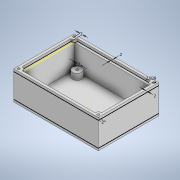
# Autodesk Inventor part: Enclosure
Saved by Autodesk Inventor 2020.2 (Build 242310000, 310)
## iProperties
Created: 2020-09-23
Part Number: Enclosure
Material: Generic
Document SubType Name: Modeling
Designer: johnf
Density: 1 g/cm^3
Appearance: Default
Author: johnf
Autodesk Inventor part; units mm, degrees
ref_plane "YZ Plane" through (0, 0, 0) normal (1, 0, 0) x (0, 1, 0)
ref_plane "XZ Plane" through (0, 0, 0) normal (0, 1, 0) x (-1, 0, 0)
ref_plane "XY Plane" through (0, 0, 0) normal (0, 0, 1) x (1, 0, 0)
sketch "Sketch1" plane through (0, 0, 0) normal (0, 1, 0) x (-1, 0, 0)
  line L0 (25, 17.5) -> (-25, 17.5) construction
  line L1 (-25, 17.5) -> (-25, -17.5) construction
  line L2 (-25, -17.5) -> (25, -17.5) construction
  line L3 (25, -17.5) -> (25, 17.5) construction
  line L4 (25, -17.5) -> (-25, 17.5) construction
  circle A0 centre (25, 17.5) radius 1
  circle A1 centre (25, -17.5) radius 1
  circle A2 centre (-25, 17.5) radius 1
  circle A3 centre (-25, -17.5) radius 1
  circle A4 centre (25, 17.5) radius 3.75
  circle A5 centre (25, -17.5) radius 3.75
  circle A6 centre (-25, -17.5) radius 3.75
  circle A7 centre (-25, 17.5) radius 3.75
  point P0 (0, 0)
  point P1 (0, 0)
  dimension "d0" = 35
  dimension "d1" = 50
  dimension "d2" = 2
  dimension "d3" = 7.5
  constraints: 10 end point, 9 coincident, 8 centre point, 6 equal radius, 2 parallel, 1 horizontal, 1 midpoint, 1 perpendicular
  measures "d0" distance of L2.end L0.start
  measures "d1" distance of L1.end L2.end
  measures "d2" diameter of A0
  measures "d3" diameter of A4
extrude "Extrusion1" add sketch "Sketch1" along normal blind 5
sketch "Sketch2" plane through (0, 0, 0) normal (0, 1, 0) x (-1, 0, 0)
  line L0 (35, -25) -> (-35, -25)
  line L1 (-35, -25) -> (-35, 25)
  line L2 (-35, 25) -> (35, 25)
  line L3 (35, 25) -> (35, -25)
  line L4 (35, 25) -> (-35, -25) construction
  line L5 (30, -22.5) -> (-30, -22.5) construction
  line L6 (-30, -22.5) -> (-30, 22.5) construction
  line L7 (-30, 22.5) -> (30, 22.5) construction
  line L8 (30, 22.5) -> (30, -22.5) construction
  line L9 (-25, -17.5) -> (25, -17.5) construction
  line L10 (25, -17.5) -> (25, 17.5) construction
  line L11 (25, 17.5) -> (-25, 17.5) construction
  line L12 (-25, 17.5) -> (-25, -17.5) construction
  line L13 (30, -22.5) -> (-30, 22.5) construction
  line L14 (-31, -21) -> (31, -21)
  line L15 (31, -21) -> (31, 21)
  line L16 (31, 21) -> (-31, 21)
  line L17 (-31, 21) -> (-31, -21)
  point P0 (0, 0)
  point P1 (0, 0)
  dimension "d6" = 70
  dimension "d7" = 60
  dimension "d8" = 45
  dimension "d9" = 5
  dimension "d10" = 50
  dimension "d11" = 4
  constraints: 36 end point, 8 parallel, 4 perpendicular, 2 horizontal, 2 midpoint, 1 coincident, 6 other
  measures "d6" distance of L0.start L0.end
  measures "d7" distance of L5.start L5.end
  measures "d8" distance of L7.end L5.start
  measures "d9" distance between parallel lines of L5 L9
  measures "d10" distance of L2.end L0.start
  measures "d11" distance between parallel lines of L3 L15
extrude "Extrusion2" add sketch "Sketch2" against normal blind 2 contours L0 L1 L2 L3 | L17 L16 L15 L14
sketch "Sketch3" plane through (0, 0, 0) normal (0, 1, 0) x (1, 0, 0)
  line L0 (-35, -25) -> (35, -25) projected
  line L1 (-35, 25) -> (35, 25)
  line L2 (35, 25) -> (35, -25)
  line L3 (35, -25) -> (-35, -25)
  line L4 (-35, -25) -> (-35, 25)
  line L5 (33, 23) -> (-33, 23)
  line L6 (-33, 23) -> (-33, -23)
  line L7 (-33, -23) -> (33, -23)
  line L8 (33, -23) -> (33, 23)
  point P0 (0, 0)
  dimension "d14" = 2
  constraints: 16 end point, 4 parallel, 2 perpendicular, 1 horizontal, 3 other
  measures "d14" distance between parallel lines of L4 L6
extrude "Extrusion3" add sketch "Sketch2" along normal blind 20
sketch "Sketch5" plane through (0, 20, 0) normal (0, 1, 0) x (1, 0, 0)
  line L0 (-35, -25) -> (-35, 25) projected
  line L1 (35, 25) -> (35, -25) projected
  line L2 (-35, 25) -> (35, 25)
  line L3 (35, 25) -> (35, -25)
  line L4 (35, -25) -> (-35, -25)
  line L5 (-35, -25) -> (-35, 25)
  line L6 (30.1716, 23) -> (-30.1716, 23)
  line L7 (-33, 20.1716) -> (-33, -20.1716)
  line L8 (-30.1716, -23) -> (30.1716, -23)
  line L9 (33, -20.1716) -> (33, 20.1716)
  line L10 (-31, 21) -> (-31, -21) projected
  arc A0 (-30.1716, -23) -> (-33, -20.1716) centre (-33, -23) ccw
  line L11 (31, 21) -> (31, -21) projected
  arc A1 (-33, 20.1716) -> (-30.1716, 23) centre (-33, 23) ccw
  arc A2 (33, -20.1716) -> (30.1716, -23) centre (33, -23) ccw
  arc A3 (30.1716, 23) -> (33, 20.1716) centre (33, 23) ccw
  point P0 (0, 0)
  dimension "d17" = 2
  dimension "d20" = 2
  dimension "d21" = 2
  dimension "d22" = 2.8284
  dimension "d23" = 2
  constraints: 16 end point, 12 point on circle, 7 point on line, 4 centre point, 4 parallel, 2 perpendicular, 1 horizontal
  measures "d17" distance between parallel lines of L2 L6
  measures "d20" distance between parallel lines of L0 L7
  measures "d21" distance between parallel lines of L3 L9
  measures "d22" radius of A3
  measures "d23" distance between parallel lines of L4 L8
extrude "Extrusion4" add sketch "Sketch5" along normal blind 2
sketch "Sketch6" plane through (0, 22, 0) normal (0, 1, 0) x (1, 0, 0)
  circle A0 centre (-33, 23) radius 1
  line L0 (-30.1716, 23) -> (30.1716, 23) projected
  line L1 (-33, -20.1716) -> (-33, 20.1716) projected
  circle A1 centre (33, 23) radius 1
  circle A2 centre (33, -23) radius 1
  circle A3 centre (-33, -23) radius 1
  line L2 (33, 20.1716) -> (33, -20.1716) projected
  line L3 (30.1716, -23) -> (-30.1716, -23) projected
  point P0 (0, 0)
  dimension "d24" = 2
  constraints: 8 point on line, 4 centre point, 3 equal radius
  measures "d24" diameter of A0
extrude "Extrusion5" cut sketch "Sketch6" against normal blind 10
body "Solid1"
